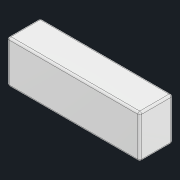
# Autodesk Inventor part: Fullymax_6s
Saved by Autodesk Inventor 2021 (Build 250183000, 183)
## iProperties
Created: 2020-09-06
Part Number: Fullymax_6s
Material: ABS プラスチック
Document SubType Name: Modeling
Designer: Yuta Kage
Mass: 300 g
Surface Area: 229.572 cm^2
Volume: 188.272 cm^3
Density: 1.06 g/cm^3
Appearance: 滑らか - 白
Author: Yuta Kage
Autodesk Inventor part; units mm, degrees
ref_plane "YZ Plane" through (0, 0, 0) normal (1, 0, 0) x (0, 1, 0)
ref_plane "XZ Plane" through (0, 0, 0) normal (0, 1, 0) x (-1, 0, 0)
ref_plane "XY Plane" through (0, 0, 0) normal (0, 0, 1) x (1, 0, 0)
sketch "スケッチ1" plane through (0, 0, 0) normal (0, 0, 1) x (1, 0, 0)
  line L0 (-70, -22.5) -> (70, -22.5)
  line L1 (70, -22.5) -> (70, 22.5)
  line L2 (70, 22.5) -> (-70, 22.5)
  line L3 (-70, 22.5) -> (-70, -22.5)
  line L4 (-70, -22.5) -> (70, 22.5) construction
  line L5 (70, -22.5) -> (-70, 22.5) construction
  point P0 (0, 0)
  dimension "d0" = 140
  dimension "d1" = 45
  constraints: 12 end point, 2 midpoint, 2 parallel, 1 horizontal, 1 perpendicular
  measures "d0" distance of L2.end L1.end
  measures "d1" distance of L1.end L0.end
extrude "押し出し1" add sketch "スケッチ1" along normal blind 35
fillet "フィレット1" radius 2 1 edges at (0, 22.5, 35)
fillet "フィレット1" radius 2 12 edges at (-70, -22.5, 17.5) (70, -22.5, 17.5) (0, -22.5, 0) (0, -22.5, 35) (-70, 22.5, 17.5) (-70, 0, 0) (-70, 0, 35) (70, 22.5, 17.5) (0, 22.5, 0) (0, 22.5, 35) (70, 0, 0) (70, 0, 35)
